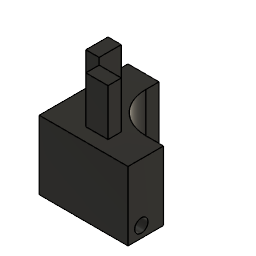
Front Base Lower (Autodesk Fusion 360 design; units mm, degrees)
Autodesk Fusion 360 part; units mm, degrees
sketch "スケッチ1" plane through (0, 0, 0) normal (0, 0, 1) x (1, 0, 0)
  line L0 (0, 0) -> (20, 0)
  line L1 (20, 0) -> (20, 20)
  line L2 (20, 20) -> (0, 20)
  line L3 (0, 20) -> (0, 0)
  constraint horizontal L0
  constraint vertical L1
  constraint horizontal L2
  constraint vertical L3
  constraint coincident L0.start L3.end
extrude "押し出し1" add sketch "スケッチ1" along normal blind 10.5
sketch "スケッチ2" plane through (0, 0, 10.5) normal (0, 0, 1) x (-1, 0, 0)
  line L0 (0, -20) -> (0, 0)
  line L1 (0, 0) -> (-20, 0)
  line L2 (-20, 0) -> (-20, -20)
  line L3 (-20, -20) -> (0, -20)
  line L4 (-7.5, -3) -> (-12.5, -3)
  line L5 (-12.5, -3) -> (-12.5, -6)
  line L6 (-12.5, -6) -> (-7.5, -6)
  line L7 (-7.5, -6) -> (-7.5, -3)
  line L8 (-6, -12.5) -> (-3, -12.5)
  line L9 (-3, -12.5) -> (-3, -7.5)
  line L10 (-3, -7.5) -> (-6, -7.5)
  line L11 (-6, -7.5) -> (-6, -12.5)
  dimension "d3" = 7.5
  dimension "d4" = 3
  dimension "d5" = 7.5
  dimension "d6" = 3
  constraint horizontal L4
  constraint vertical L5
  constraint horizontal L6
  constraint vertical L7
  constraint horizontal L8
  constraint vertical L9
  constraint horizontal L10
  constraint vertical L11
  measures "d3" distance of L3 L8
  measures "d4" distance of L0 L9
  measures "d5" distance of L0 L7
  measures "d6" distance of L1 L4
extrude "押し出し2" add sketch "スケッチ2" along normal blind 10.5 contours L4 L5 L6 L7 | L8 L9 L10 L11
sketch "スケッチ4" plane through (0, 0, 0) normal (0, 0, -1) x (1, 0, 0)
  line L0 (0, 0) -> (0, -20)
  line L1 (0, -20) -> (20, -20)
  line L2 (20, -20) -> (20, 0)
  line L3 (20, 0) -> (0, 0)
  line L4 (20, -20) -> (7, -20)
  line L5 (7, -20) -> (7, -8)
  line L6 (7, -8) -> (20, -8)
  line L7 (20, -8) -> (20, -20)
  dimension "d14" = 12
  dimension "d15" = 13
  constraint horizontal L4
  constraint vertical L5
  constraint horizontal L6
  constraint vertical L7
  constraint coincident L1.end L2.start
  measures "d14" distance of L1.end L6.end
  measures "d15" distance of L1.end L4.end
extrude "押し出し4" cut sketch "スケッチ4" against normal blind 18 contours L1 L2 L4 L5 L6 L7
fillet "フィレット1" radius 9 1 edges at (7, 8, 5.25)
extrude "押し出し5" add 1 faces at (11.1548, 2.7882, 0) along direction (0, 0, -1) blind 5
sketch "スケッチ3" plane through (20, 0, 0) normal (1, 0, 0) x (0, 1, 0)
  line L0 (8, 10.5) -> (0, 10.5)
  line L1 (0, 10.5) -> (0, -5)
  circle A0 centre (3, -2.5) radius 1.5
  line L2 (8, -5) -> (8, 10.5)
  line L3 (0, -5) -> (8, -5)
  dimension "d9" = 3
  dimension "d10" = 3
  dimension "d22" = 2.5
  measures "d9" diameter of A0
  measures "d10" distance of L1 A0.centre
  measures "d22" distance of A0.centre L3
extrude "押し出し3" cut sketch "スケッチ3" against normal blind 22 contours A0
